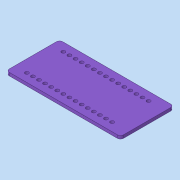
# Autodesk Inventor part: BackupNanoCasePart2
Saved by Autodesk Inventor 2017 (Build 210142000, 142)
## iProperties
Created: 2018-02-21
Part Number: BackupNanoCasePart2
Material: ABS Plastic
Document SubType Name: Modeling
Designer: Derek Wider
Density: 1.06 g/cm^3
Appearance: Violet
Author: Derek Wider
Autodesk Inventor part; units mm, degrees
ref_plane "YZ Plane" through (0, 0, 0) normal (1, 0, 0) x (0, 1, 0)
ref_plane "XZ Plane" through (0, 0, 0) normal (0, 1, 0) x (-1, 0, 0)
ref_plane "XY Plane" through (0, 0, 0) normal (0, 0, 1) x (1, 0, 0)
sketch "Sketch1" plane through (0, 0, 0) normal (0, 1, 0) x (-1, 0, 0)
  line L0 (0, 0) -> (47.625, 0)
  line L1 (47.625, 0) -> (47.625, -22.225)
  line L2 (47.625, -22.225) -> (0, -22.225)
  line L3 (0, -22.225) -> (0, 0)
  dimension "d0" = 22.225
  dimension "d1" = 47.625
  constraints: 8 end point, 2 parallel, 1 horizontal, 1 perpendicular
  measures "d0" distance of L2.end L0.start
  measures "d1" distance of L1.end L2.end
extrude "Extrusion1" add sketch "Sketch1" along normal blind 1.27
sketch "Sketch2" plane through (0, 1.27, 0) normal (0, 1, 0) x (1, 0, 0)
  circle A0 centre (-6.985, 3.4925) radius 0.762
  line L0 (-47.625, 0) -> (0, 0) construction
  line L1 (0, 0) -> (0, 22.225) construction
  line L2 (0, 22.225) -> (-47.625, 22.225) construction
  line L3 (-47.625, 22.225) -> (-47.625, 0) construction
  circle A1 centre (-9.525, 3.4925) radius 0.762
  circle A2 centre (-12.065, 3.4925) radius 0.762
  circle A3 centre (-14.605, 3.4925) radius 0.762
  circle A4 centre (-17.145, 3.4925) radius 0.762
  circle A5 centre (-19.685, 3.4925) radius 0.762
  circle A6 centre (-22.225, 3.4925) radius 0.762
  circle A7 centre (-24.765, 3.4925) radius 0.762
  circle A8 centre (-27.305, 3.4925) radius 0.762
  circle A9 centre (-29.845, 3.4925) radius 0.762
  circle A10 centre (-32.385, 3.4925) radius 0.762
  circle A11 centre (-34.925, 3.4925) radius 0.762
  circle A12 centre (-37.465, 3.4925) radius 0.762
  circle A13 centre (-40.005, 3.4925) radius 0.762
  circle A14 centre (-42.545, 3.4925) radius 0.762
  circle A15 centre (-6.985, 18.7325) radius 0.762
  circle A16 centre (-9.525, 18.7325) radius 0.762
  circle A17 centre (-12.065, 18.7325) radius 0.762
  circle A18 centre (-14.605, 18.7325) radius 0.762
  circle A19 centre (-17.145, 18.7325) radius 0.762
  circle A20 centre (-19.685, 18.7325) radius 0.762
  circle A21 centre (-22.225, 18.7325) radius 0.762
  circle A22 centre (-24.765, 18.7325) radius 0.762
  circle A23 centre (-27.305, 18.7325) radius 0.762
  circle A24 centre (-29.845, 18.7325) radius 0.762
  circle A25 centre (-32.385, 18.7325) radius 0.762
  circle A26 centre (-34.925, 18.7325) radius 0.762
  circle A27 centre (-37.465, 18.7325) radius 0.762
  circle A28 centre (-40.005, 18.7325) radius 0.762
  circle A29 centre (-42.545, 18.7325) radius 0.762
  dimension "d4" = 1.524
  dimension "d5" = 3.4925
  dimension "d6" = 6.985
  dimension "d9" = 2.54
  dimension "d12" = 15.24
  constraints: 30 centre point, 1 horizontal, 1 vertical, 58 other
  measures "d4" diameter of A0
  measures "d5" vertical distance of point (0, 0) A0.centre
  measures "d6" horizontal distance of point (0, 0) A0.centre
  measures "d9" distance of A0.centre A1.centre
  measures "d12" distance of A0.centre A15.centre
extrude "Extrusion2" cut sketch "Sketch2" against normal through all
fillet "Fillet1" radius 1.27 4 edges at (-47.625, 0.635, 0) (-47.625, 0.635, -22.225) (0, 0.635, 0) (0, 0.635, -22.225)
body "Solid1"
